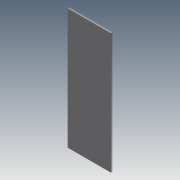
# Autodesk Inventor part: small
Saved by Autodesk Inventor 2011 (Build 150239000, 239)
## iProperties
Created: 2011-01-01
Part Number: small
Document SubType Name: Modeling
Designer: Matthew
Density: 1 g/cm^3
Author: Matthew
Autodesk Inventor part; units mm, degrees
ref_plane "YZ Plane" through (0, 0, 0) normal (1, 0, 0) x (0, 1, 0)
ref_plane "XZ Plane" through (0, 0, 0) normal (0, 1, 0) x (-1, 0, 0)
ref_plane "XY Plane" through (0, 0, 0) normal (0, 0, 1) x (1, 0, 0)
sketch "Sketch1" plane through (0, 0, 0) normal (0, 0, 1) x (1, 0, 0)
  line L0 (-32.8778, 15.3939) -> (140.0962, 15.3939)
  line L1 (140.0962, 15.3939) -> (140.0962, -466.4441)
  line L2 (140.0962, -466.4441) -> (-32.8778, -466.4441)
  line L3 (-32.8778, -466.4441) -> (-32.8778, 15.3939)
  point P0 (0, 0)
  dimension "d0" = 172.974
  dimension "d1" = 481.838
  constraints: 8 end point, 2 parallel, 1 horizontal, 1 perpendicular
  measures "d0" distance of L1.end L2.end
  measures "d1" distance of L0.end L1.end
extrude "Extrusion1" add sketch "Sketch1" along normal blind 6.35
body "Solid1"
